Autodesk Inventor part; units mm, degrees
(part 2 of 2)
  point P155 (-22.7596, 134.1998)
  point P156 (-16.0635, 134.1998)
  point P157 (-9.3673, 134.1998)
  point P158 (-2.6712, 134.1998)
  point P159 (-36.1519, 134.1998)
  point P160 (-36.1519, 137.1998)
  point P161 (-32.8038, 140.1998)
  point P162 (-29.4558, 137.1998)
  point P163 (-26.8577, 132.6998)
  point P164 (-26.1077, 140.1998)
  point P165 (-19.4115, 140.1998)
  point P166 (-12.7154, 140.1998)
  point P167 (-6.0192, 140.1998)
  point P168 (-39.5, 140.1998)
  point P169 (-2.5841, 26.25)
  point P170 (-9.2803, 26.25)
  point P171 (-22.6726, 26.25)
  point P172 (-15.9764, 26.25)
  point P173 (-29.3688, 26.25)
  point P174 (-36.0649, 26.25)
  point P175 (-5.9322, 29.25)
  point P176 (0.7639, 29.25)
  point P177 (-29.3688, 29.25)
  point P178 (-22.6726, 29.25)
  point P179 (-19.3245, 29.25)
  point P180 (-12.6284, 29.25)
  point P181 (-26.0207, 29.25)
  point P182 (-32.7168, 29.25)
  point P183 (-2.6712, 14.25)
  point P184 (-9.3673, 14.25)
  point P185 (-22.7596, 14.25)
  point P186 (-16.0635, 14.25)
  point P187 (-29.4558, 14.25)
  point P188 (-36.1519, 14.25)
  point P189 (-6.0192, 17.25)
  point P190 (0.6769, 17.25)
  point P191 (-29.4558, 17.25)
  point P192 (-22.7596, 17.25)
  point P193 (-12.7154, 17.25)
  point P194 (-26.1077, 17.25)
  point P195 (-32.8038, 17.25)
  point P196 (-38.65, 118.709)
  point P197 (-38.65, 113.6905)
  point P198 (-38.65, 137.7905)
  point P199 (-38.65, 17.7407)
  dimension "d0" = 0.35
  dimension "d1" = 2
  constraints: 1624 end point, 3 horizontal, 3 parallel, 3 vertical, 1 perpendicular, 1799 other
  measures "d1" distance between parallel lines of L13 L16
extrude "Extrusión1" add sketch "Boceto1" along normal blind 5 contours L14 L13 L12 L605 L608 L17 L568 L567 L569 L496 L495 L497 L424 L423 L425 L352 L351 L353 L280 L279 L281 L208 L207 L209 L136 L135 L137 L783 L782 L780 L25 L24 L23 L16 L22 L35 L34 L798 L801 L812 L805 L810 L790 L19 L18 L752 L749 L15 | L749 L752 L17 L712 L711 L713 L679 L676 L12 | L676 L679 L17 L680 L677 L12 | L677 L680 L17 L640 L639 L641 L607 L604 L12 | L752 L750 L751 L18 L721 L720 L719 L718 L717 L722 L724 L723 L728 L727 L726 L725 L732 L731 L729 L734 L730 L733 L738 L737 L735 L740 L736 L739 L744 L743 L741 L746 L742 L745 L19 L708 L707 L705 L636 L635 L633 L564 L563 L561 L492 L491 L489 L420 L419 L417 L348 L347 L345 L276 L275 L273 L204 L203 L201 L132 L131 L129 L758 L756 L753 L794 L792 L789 L16 L790 L797 L795 L811 L809 L810 L805 L807 L808 L806 L804 L812 L801 L803 L802 L800 L799 L798 L34 L33 L38 L37 L36 L35 L22 L21 L20 L25 L17 L68 L64 L67 L780 L778 L781 L784 L783 L104 L102 L103 L137 L140 L138 L139 L136 L176 L174 L175 L209 L212 L210 L211 L208 L248 L246 L247 L281 L284 L282 L283 L280 L320 L318 L319 L353 L356 L354 L355 L352 L392 L390 L391 L425 L428 L426 L427 L424 L464 L462 L463 L497 L500 L498 L499 L496 L536 L534 L535 L569 L572 L570 L571 L568 L608 L606 L607 L641 L644 L642 L643 L640 L680 L678 L679 L713 L716 L714 L715 L712 | L604 L607 L17 L608 L605 L12 | L17 L713 L711 L712 | L17 L641 L639 L640 | L17 L569 L567 L568 | L17 L497 L495 L496 | L17 L425 L423 L424 | L17 L353 L351 L352 | L17 L281 L279 L280 | L17 L209 L207 L208 | L17 L137 L135 L136 | L17 L23 L24 L25 | L23 L16 L17 | L16 L22 L23
sketch "Boceto2" plane through (0, 0, 5) normal (0, 0, 1) x (1, 0, 0)
  line L0 (-40.65, 9.35) -> (-1.35, 9.35) projected
  line L1 (-1.35, 9.35) -> (-1.35, 144.35) projected
  line L2 (-1.35, 144.35) -> (-40.65, 144.35) projected
  line L3 (-40.65, 144.35) -> (-40.65, 9.35) projected
  line L4 (-38.65, 118.709) -> (-36.9019, 117.6998) projected
  line L5 (-36.9019, 117.6998) -> (-36.9019, 114.6998) projected
  line L6 (-36.9019, 114.6998) -> (-38.65, 113.6905) projected
  line L7 (-38.65, 113.6905) -> (-38.65, 118.709) projected
  line L8 (-38.65, 137.7905) -> (-38.65, 142.35) projected
  line L9 (-38.65, 142.35) -> (-38.2014, 142.35) projected
  line L10 (-38.2014, 142.35) -> (-36.9885, 141.6498) projected
  line L11 (-36.9885, 141.6498) -> (-36.9885, 138.7498) projected
  line L12 (-36.9885, 138.7498) -> (-38.65, 137.7905) projected
  line L13 (-38.65, 22.7593) -> (-36.9019, 21.75) projected
  line L14 (-36.9019, 21.75) -> (-36.9019, 18.75) projected
  line L15 (-36.9019, 18.75) -> (-38.65, 17.7407) projected
  line L16 (-38.65, 17.7407) -> (-38.65, 22.7593) projected
  line L17 (-38.65, 29.6905) -> (-38.65, 34.709) projected
  line L18 (-38.65, 34.709) -> (-36.9019, 33.6998) projected
  line L19 (-36.9019, 33.6998) -> (-36.9019, 30.6998) projected
  line L20 (-36.9019, 30.6998) -> (-38.65, 29.6905) projected
  line L21 (-38.65, 36.642) -> (-38.65, 39.7575) projected
  line L22 (-38.65, 39.7575) -> (-36.1519, 41.1998) projected
  line L23 (-36.1519, 41.1998) -> (-33.5538, 39.6998) projected
  line L24 (-33.5538, 39.6998) -> (-33.5538, 36.6998) projected
  line L25 (-33.5538, 36.6998) -> (-36.1519, 35.1998) projected
  line L26 (-36.1519, 35.1998) -> (-38.65, 36.642) projected
  line L27 (-38.65, 41.6905) -> (-38.65, 46.709) projected
  line L28 (-38.65, 46.709) -> (-36.9019, 45.6998) projected
  line L29 (-36.9019, 45.6998) -> (-36.9019, 42.6998) projected
  line L30 (-36.9019, 42.6998) -> (-38.65, 41.6905) projected
  line L31 (-38.65, 48.642) -> (-38.65, 51.7575) projected
  line L32 (-38.65, 51.7575) -> (-36.1519, 53.1998) projected
  line L33 (-36.1519, 53.1998) -> (-33.5538, 51.6998) projected
  line L34 (-33.5538, 51.6998) -> (-33.5538, 48.6998) projected
  line L35 (-33.5538, 48.6998) -> (-36.1519, 47.1998) projected
  line L36 (-36.1519, 47.1998) -> (-38.65, 48.642) projected
  line L37 (-38.65, 53.6905) -> (-38.65, 58.709) projected
  line L38 (-38.65, 58.709) -> (-36.9019, 57.6998) projected
  line L39 (-36.9019, 57.6998) -> (-36.9019, 54.6998) projected
  line L40 (-36.9019, 54.6998) -> (-38.65, 53.6905) projected
  line L41 (-38.65, 60.642) -> (-38.65, 63.7575) projected
  line L42 (-38.65, 63.7575) -> (-36.1519, 65.1998) projected
  line L43 (-36.1519, 65.1998) -> (-33.5538, 63.6998) projected
  line L44 (-33.5538, 63.6998) -> (-33.5538, 60.6998) projected
  line L45 (-33.5538, 60.6998) -> (-36.1519, 59.1998) projected
  line L46 (-36.1519, 59.1998) -> (-38.65, 60.642) projected
  line L47 (-38.65, 65.6905) -> (-38.65, 70.709) projected
  line L48 (-38.65, 70.709) -> (-36.9019, 69.6998) projected
  line L49 (-36.9019, 69.6998) -> (-36.9019, 66.6998) projected
  line L50 (-36.9019, 66.6998) -> (-38.65, 65.6905) projected
  line L51 (-38.65, 72.642) -> (-38.65, 75.7575) projected
  line L52 (-38.65, 75.7575) -> (-36.1519, 77.1998) projected
  line L53 (-36.1519, 77.1998) -> (-33.5538, 75.6998) projected
  line L54 (-33.5538, 75.6998) -> (-33.5538, 72.6998) projected
  line L55 (-33.5538, 72.6998) -> (-36.1519, 71.1998) projected
  line L56 (-36.1519, 71.1998) -> (-38.65, 72.642) projected
  line L57 (-38.65, 77.6905) -> (-38.65, 82.709) projected
  line L58 (-38.65, 82.709) -> (-36.9019, 81.6998) projected
  line L59 (-36.9019, 81.6998) -> (-36.9019, 78.6998) projected
  line L60 (-36.9019, 78.6998) -> (-38.65, 77.6905) projected
  line L61 (-38.65, 84.642) -> (-38.65, 87.7575) projected
  line L62 (-38.65, 87.7575) -> (-36.1519, 89.1998) projected
  line L63 (-36.1519, 89.1998) -> (-33.5538, 87.6998) projected
  line L64 (-33.5538, 87.6998) -> (-33.5538, 84.6998) projected
  line L65 (-33.5538, 84.6998) -> (-36.1519, 83.1998) projected
  line L66 (-36.1519, 83.1998) -> (-38.65, 84.642) projected
  line L67 (-38.65, 89.6905) -> (-38.65, 94.709) projected
  line L68 (-38.65, 94.709) -> (-36.9019, 93.6998) projected
  line L69 (-36.9019, 93.6998) -> (-36.9019, 90.6998) projected
  line L70 (-36.9019, 90.6998) -> (-38.65, 89.6905) projected
  line L71 (-38.65, 96.642) -> (-38.65, 99.7575) projected
  line L72 (-38.65, 99.7575) -> (-36.1519, 101.1998) projected
  line L73 (-36.1519, 101.1998) -> (-33.5538, 99.6998) projected
  line L74 (-33.5538, 99.6998) -> (-33.5538, 96.6998) projected
  line L75 (-33.5538, 96.6998) -> (-36.1519, 95.1998) projected
  line L76 (-36.1519, 95.1998) -> (-38.65, 96.642) projected
  line L77 (-38.65, 101.6905) -> (-38.65, 106.709) projected
  line L78 (-38.65, 106.709) -> (-36.9019, 105.6998) projected
  line L79 (-36.9019, 105.6998) -> (-36.9019, 102.6998) projected
  line L80 (-36.9019, 102.6998) -> (-38.65, 101.6905) projected
  line L81 (-38.65, 108.642) -> (-38.65, 111.7575) projected
  line L82 (-38.65, 111.7575) -> (-36.1519, 113.1998) projected
  line L83 (-36.1519, 113.1998) -> (-33.5538, 111.6998) projected
  line L84 (-33.5538, 111.6998) -> (-33.5538, 108.6998) projected
  line L85 (-33.5538, 108.6998) -> (-36.1519, 107.1998) projected
  line L86 (-36.1519, 107.1998) -> (-38.65, 108.642) projected
  line L87 (-38.65, 125.6905) -> (-38.65, 130.709) projected
  line L88 (-38.65, 130.709) -> (-36.9019, 129.6998) projected
  line L89 (-36.9019, 129.6998) -> (-36.9019, 126.6998) projected
  line L90 (-36.9019, 126.6998) -> (-38.65, 125.6905) projected
  line L91 (-38.65, 120.642) -> (-38.65, 123.7575) projected
  line L92 (-38.65, 123.7575) -> (-36.1519, 125.1998) projected
  line L93 (-36.1519, 125.1998) -> (-33.5538, 123.6998) projected
  line L94 (-33.5538, 123.6998) -> (-33.5538, 120.6998) projected
  line L95 (-33.5538, 120.6998) -> (-36.1519, 119.1998) projected
  line L96 (-36.1519, 119.1998) -> (-38.65, 120.642) projected
  line L97 (-38.65, 132.642) -> (-38.65, 135.7575) projected
  line L98 (-38.65, 135.7575) -> (-36.1519, 137.1998) projected
  line L99 (-36.1519, 137.1998) -> (-33.5538, 135.6998) projected
  line L100 (-33.5538, 135.6998) -> (-33.5538, 132.6998) projected
  line L101 (-33.5538, 132.6998) -> (-36.1519, 131.1998) projected
  line L102 (-36.1519, 131.1998) -> (-38.65, 132.642) projected
  line L103 (-34.1025, 142.35) -> (-31.5052, 142.35) projected
  line L104 (-31.5052, 142.35) -> (-30.2924, 141.6498) projected
  line L105 (-30.2924, 141.6498) -> (-30.2924, 138.7498) projected
  line L106 (-30.2924, 138.7498) -> (-32.8038, 137.2998) projected
  line L107 (-32.8038, 137.2998) -> (-35.3153, 138.7498) projected
  line L108 (-35.3153, 138.7498) -> (-35.3153, 141.6498) projected
  line L109 (-35.3153, 141.6498) -> (-34.1025, 142.35) projected
  line L110 (-27.4063, 142.35) -> (-24.8091, 142.35) projected
  line L111 (-24.8091, 142.35) -> (-23.5962, 141.6498) projected
  line L112 (-23.5962, 141.6498) -> (-23.5962, 138.7498) projected
  line L113 (-23.5962, 138.7498) -> (-26.1077, 137.2998) projected
  line L114 (-26.1077, 137.2998) -> (-28.6192, 138.7498) projected
  line L115 (-28.6192, 138.7498) -> (-28.6192, 141.6498) projected
  line L116 (-28.6192, 141.6498) -> (-27.4063, 142.35) projected
  line L117 (-20.7102, 142.35) -> (-18.1129, 142.35) projected
  line L118 (-18.1129, 142.35) -> (-16.9001, 141.6498) projected
  line L119 (-16.9001, 141.6498) -> (-16.9001, 138.7498) projected
  line L120 (-16.9001, 138.7498) -> (-19.4115, 137.2998) projected
  line L121 (-19.4115, 137.2998) -> (-21.923, 138.7498) projected
  line L122 (-21.923, 138.7498) -> (-21.923, 141.6498) projected
  line L123 (-21.923, 141.6498) -> (-20.7102, 142.35) projected
  line L124 (-14.014, 142.35) -> (-11.4168, 142.35) projected
  line L125 (-11.4168, 142.35) -> (-10.2039, 141.6498) projected
  line L126 (-10.2039, 141.6498) -> (-10.2039, 138.7498) projected
  line L127 (-10.2039, 138.7498) -> (-12.7154, 137.2998) projected
  line L128 (-12.7154, 137.2998) -> (-15.2269, 138.7498) projected
  line L129 (-15.2269, 138.7498) -> (-15.2269, 141.6498) projected
  line L130 (-15.2269, 141.6498) -> (-14.014, 142.35) projected
  line L131 (-7.3179, 142.35) -> (-4.7206, 142.35) projected
  line L132 (-4.7206, 142.35) -> (-3.5078, 141.6498) projected
  line L133 (-3.5078, 141.6498) -> (-3.5078, 138.7498) projected
  line L134 (-3.5078, 138.7498) -> (-6.0192, 137.2998) projected
  line L135 (-6.0192, 137.2998) -> (-8.5307, 138.7498) projected
  line L136 (-8.5307, 138.7498) -> (-8.5307, 141.6498) projected
  line L137 (-8.5307, 141.6498) -> (-7.3179, 142.35) projected
  line L138 (-3.35, 136.8078) -> (-3.35, 131.5917) projected
  line L139 (-3.35, 131.5917) -> (-5.2692, 132.6998) projected
  line L140 (-5.2692, 132.6998) -> (-5.2692, 135.6998) projected
  line L141 (-5.2692, 135.6998) -> (-3.35, 136.8078) projected
  line L142 (-3.35, 124.8078) -> (-3.35, 119.5917) projected
  line L143 (-3.35, 119.5917) -> (-5.2692, 120.6998) projected
  line L144 (-5.2692, 120.6998) -> (-5.2692, 123.6998) projected
  line L145 (-5.2692, 123.6998) -> (-3.35, 124.8078) projected
  line L146 (-3.35, 112.8078) -> (-3.35, 107.5917) projected
  line L147 (-3.35, 107.5917) -> (-5.2692, 108.6998) projected
  line L148 (-5.2692, 108.6998) -> (-5.2692, 111.6998) projected
  line L149 (-5.2692, 111.6998) -> (-3.35, 112.8078) projected
  line L150 (-3.35, 100.8078) -> (-3.35, 95.5917) projected
  line L151 (-3.35, 95.5917) -> (-5.2692, 96.6998) projected
  line L152 (-5.2692, 96.6998) -> (-5.2692, 99.6998) projected
  line L153 (-5.2692, 99.6998) -> (-3.35, 100.8078) projected
  line L154 (-3.35, 88.8078) -> (-3.35, 83.5917) projected
  line L155 (-3.35, 83.5917) -> (-5.2692, 84.6998) projected
  line L156 (-5.2692, 84.6998) -> (-5.2692, 87.6998) projected
  line L157 (-5.2692, 87.6998) -> (-3.35, 88.8078) projected
  line L158 (-3.35, 76.8078) -> (-3.35, 71.5917) projected
  line L159 (-3.35, 71.5917) -> (-5.2692, 72.6998) projected
  line L160 (-5.2692, 72.6998) -> (-5.2692, 75.6998) projected
  line L161 (-5.2692, 75.6998) -> (-3.35, 76.8078) projected
  line L162 (-3.35, 64.8078) -> (-3.35, 59.5917) projected
  line L163 (-3.35, 59.5917) -> (-5.2692, 60.6998) projected
  line L164 (-5.2692, 60.6998) -> (-5.2692, 63.6998) projected
  line L165 (-5.2692, 63.6998) -> (-3.35, 64.8078) projected
  line L166 (-3.35, 52.8078) -> (-3.35, 47.5917) projected
  line L167 (-3.35, 47.5917) -> (-5.2692, 48.6998) projected
  line L168 (-5.2692, 48.6998) -> (-5.2692, 51.6998) projected
  line L169 (-5.2692, 51.6998) -> (-3.35, 52.8078) projected
  line L170 (-3.35, 40.8078) -> (-3.35, 35.5917) projected
  line L171 (-3.35, 35.5917) -> (-5.2692, 36.6998) projected
  line L172 (-5.2692, 36.6998) -> (-5.2692, 39.6998) projected
  line L173 (-5.2692, 39.6998) -> (-3.35, 40.8078) projected
  line L174 (-3.35, 28.8078) -> (-3.35, 23.6922) projected
  line L175 (-3.35, 23.6922) -> (-5.1822, 24.75) projected
  line L176 (-5.1822, 24.75) -> (-5.1822, 27.75) projected
  line L177 (-5.1822, 27.75) -> (-3.35, 28.8078) projected
  line L178 (-3.35, 16.8581) -> (-3.35, 11.6419) projected
  line L179 (-3.35, 11.6419) -> (-5.2692, 12.75) projected
  line L180 (-5.2692, 12.75) -> (-5.2692, 15.75) projected
  line L181 (-5.2692, 15.75) -> (-3.35, 16.8581) projected
  line L182 (-9.3673, 11.25) -> (-11.9654, 12.75) projected
  line L183 (-11.9654, 12.75) -> (-11.9654, 15.75) projected
  line L184 (-11.9654, 15.75) -> (-9.3673, 17.25) projected
  line L185 (-9.3673, 17.25) -> (-6.7692, 15.75) projected
  line L186 (-6.7692, 15.75) -> (-6.7692, 12.75) projected
  line L187 (-6.7692, 12.75) -> (-9.3673, 11.25) projected
  line L188 (-16.0635, 11.25) -> (-18.6615, 12.75) projected
  line L189 (-18.6615, 12.75) -> (-18.6615, 15.75) projected
  line L190 (-18.6615, 15.75) -> (-16.0635, 17.25) projected
  line L191 (-16.0635, 17.25) -> (-13.4654, 15.75) projected
  line L192 (-13.4654, 15.75) -> (-13.4654, 12.75) projected
  line L193 (-13.4654, 12.75) -> (-16.0635, 11.25) projected
  line L194 (-22.7596, 11.25) -> (-25.3577, 12.75) projected
  line L195 (-25.3577, 12.75) -> (-25.3577, 15.75) projected
  line L196 (-25.3577, 15.75) -> (-22.7596, 17.25) projected
  line L197 (-22.7596, 17.25) -> (-20.1615, 15.75) projected
  line L198 (-20.1615, 15.75) -> (-20.1615, 12.75) projected
  line L199 (-20.1615, 12.75) -> (-22.7596, 11.25) projected
  line L200 (-29.4558, 11.25) -> (-32.0538, 12.75) projected
  line L201 (-32.0538, 12.75) -> (-32.0538, 15.75) projected
  line L202 (-32.0538, 15.75) -> (-29.4558, 17.25) projected
  line L203 (-29.4558, 17.25) -> (-26.8577, 15.75) projected
  line L204 (-26.8577, 15.75) -> (-26.8577, 12.75) projected
  line L205 (-26.8577, 12.75) -> (-29.4558, 11.25) projected
  line L206 (-36.3251, 11.35) -> (-38.65, 12.6923) projected
  line L207 (-38.65, 12.6923) -> (-38.65, 15.8077) projected
  line L208 (-38.65, 15.8077) -> (-36.1519, 17.25) projected
  line L209 (-36.1519, 17.25) -> (-33.5538, 15.75) projected
  line L210 (-33.5538, 15.75) -> (-33.5538, 12.75) projected
  line L211 (-33.5538, 12.75) -> (-35.9787, 11.35) projected
  line L212 (-9.2803, 29.25) -> (-6.6822, 27.75) projected
  line L213 (-6.6822, 27.75) -> (-6.6822, 24.75) projected
  line L214 (-6.6822, 24.75) -> (-9.2803, 23.25) projected
  line L215 (-9.2803, 23.25) -> (-11.8784, 24.75) projected
  line L216 (-11.8784, 24.75) -> (-11.8784, 27.75) projected
  line L217 (-11.8784, 27.75) -> (-9.2803, 29.25) projected
  line L218 (-18.5745, 24.75) -> (-18.5745, 27.75) projected
  line L219 (-18.5745, 27.75) -> (-15.9764, 29.25) projected
  line L220 (-15.9764, 29.25) -> (-13.3784, 27.75) projected
  line L221 (-13.3784, 27.75) -> (-13.3784, 24.75) projected
  line L222 (-13.3784, 24.75) -> (-15.9764, 23.25) projected
  line L223 (-15.9764, 23.25) -> (-18.5745, 24.75) projected
  line L224 (-22.6726, 23.25) -> (-25.2707, 24.75) projected
  line L225 (-25.2707, 24.75) -> (-25.2707, 27.75) projected
  line L226 (-25.2707, 27.75) -> (-22.6726, 29.25) projected
  line L227 (-22.6726, 29.25) -> (-20.0745, 27.75) projected
  line L228 (-20.0745, 27.75) -> (-20.0745, 24.75) projected
  line L229 (-20.0745, 24.75) -> (-22.6726, 23.25) projected
  line L230 (-29.3688, 23.25) -> (-31.9668, 24.75) projected
  line L231 (-31.9668, 24.75) -> (-31.9668, 27.75) projected
  line L232 (-31.9668, 27.75) -> (-29.3688, 29.25) projected
  line L233 (-29.3688, 29.25) -> (-26.7707, 27.75) projected
  line L234 (-26.7707, 27.75) -> (-26.7707, 24.75) projected
  line L235 (-26.7707, 24.75) -> (-29.3688, 23.25) projected
  line L236 (-36.0649, 23.25) -> (-38.663, 24.75) projected
  line L237 (-38.663, 24.75) -> (-38.663, 27.75) projected
  line L238 (-38.663, 27.75) -> (-36.0649, 29.25) projected
  line L239 (-36.0649, 29.25) -> (-33.4668, 27.75) projected
  line L240 (-33.4668, 27.75) -> (-33.4668, 24.75) projected
  line L241 (-33.4668, 24.75) -> (-36.0649, 23.25) projected
  line L242 (-29.4558, 131.1998) -> (-32.0538, 132.6998) projected
  line L243 (-32.0538, 132.6998) -> (-32.0538, 135.6998) projected
  line L244 (-32.0538, 135.6998) -> (-29.4558, 137.1998) projected
  line L245 (-29.4558, 137.1998) -> (-26.8577, 135.6998) projected
  line L246 (-26.8577, 135.6998) -> (-26.8577, 132.6998) projected
  line L247 (-26.8577, 132.6998) -> (-29.4558, 131.1998) projected
  line L248 (-18.6615, 132.6998) -> (-18.6615, 135.6998) projected
  line L249 (-18.6615, 135.6998) -> (-16.0635, 137.1998) projected
  line L250 (-16.0635, 137.1998) -> (-13.4654, 135.6998) projected
  line L251 (-13.4654, 135.6998) -> (-13.4654, 132.6998) projected
  line L252 (-13.4654, 132.6998) -> (-16.0635, 131.1998) projected
  line L253 (-16.0635, 131.1998) -> (-18.6615, 132.6998) projected
  line L254 (-22.7596, 131.1998) -> (-25.3577, 132.6998) projected
  line L255 (-25.3577, 132.6998) -> (-25.3577, 135.6998) projected
  line L256 (-25.3577, 135.6998) -> (-22.7596, 137.1998) projected
  line L257 (-22.7596, 137.1998) -> (-20.1615, 135.6998) projected
  line L258 (-20.1615, 135.6998) -> (-20.1615, 132.6998) projected
  line L259 (-20.1615, 132.6998) -> (-22.7596, 131.1998) projected
  line L260 (-6.7692, 132.6998) -> (-9.3673, 131.1998) projected
  line L261 (-9.3673, 131.1998) -> (-11.9654, 132.6998) projected
  line L262 (-11.9654, 132.6998) -> (-11.9654, 135.6998) projected
  line L263 (-11.9654, 135.6998) -> (-9.3673, 137.1998) projected
  line L264 (-9.3673, 137.1998) -> (-6.7692, 135.6998) projected
  line L265 (-6.7692, 135.6998) -> (-6.7692, 132.6998) projected
  line L266 (-32.8038, 125.1998) -> (-35.4019, 126.6998) projected
  line L267 (-35.4019, 126.6998) -> (-35.4019, 129.6998) projected
  line L268 (-35.4019, 129.6998) -> (-32.8038, 131.1998) projected
  line L269 (-32.8038, 131.1998) -> (-30.2058, 129.6998) projected
  line L270 (-30.2058, 129.6998) -> (-30.2058, 126.6998) projected
  line L271 (-30.2058, 126.6998) -> (-32.8038, 125.1998) projected
  line L272 (-22.0096, 126.6998) -> (-22.0096, 129.6998) projected
  line L273 (-22.0096, 129.6998) -> (-19.4115, 131.1998) projected
  line L274 (-19.4115, 131.1998) -> (-16.8135, 129.6998) projected
  line L275 (-16.8135, 129.6998) -> (-16.8135, 126.6998) projected
  line L276 (-16.8135, 126.6998) -> (-19.4115, 125.1998) projected
  line L277 (-19.4115, 125.1998) -> (-22.0096, 126.6998) projected
  line L278 (-26.1077, 125.1998) -> (-28.7058, 126.6998) projected
  line L279 (-28.7058, 126.6998) -> (-28.7058, 129.6998) projected
  line L280 (-28.7058, 129.6998) -> (-26.1077, 131.1998) projected
  line L281 (-26.1077, 131.1998) -> (-23.5096, 129.6998) projected
  line L282 (-23.5096, 129.6998) -> (-23.5096, 126.6998) projected
  line L283 (-23.5096, 126.6998) -> (-26.1077, 125.1998) projected
  line L284 (-10.1173, 126.6998) -> (-12.7154, 125.1998) projected
  line L285 (-12.7154, 125.1998) -> (-15.3135, 126.6998) projected
  line L286 (-15.3135, 126.6998) -> (-15.3135, 129.6998) projected
  line L287 (-15.3135, 129.6998) -> (-12.7154, 131.1998) projected
  line L288 (-12.7154, 131.1998) -> (-10.1173, 129.6998) projected
  line L289 (-10.1173, 129.6998) -> (-10.1173, 126.6998) projected
  line L290 (-6.0192, 125.1998) -> (-8.6173, 126.6998) projected
  line L291 (-8.6173, 126.6998) -> (-8.6173, 129.6998) projected
  line L292 (-8.6173, 129.6998) -> (-6.0192, 131.1998) projected
  line L293 (-6.0192, 131.1998) -> (-3.4212, 129.6998) projected
  line L294 (-3.4212, 129.6998) -> (-3.4212, 126.6998) projected
  line L295 (-3.4212, 126.6998) -> (-6.0192, 125.1998) projected
  line L296 (-29.4558, 119.1998) -> (-32.0538, 120.6998) projected
  line L297 (-32.0538, 120.6998) -> (-32.0538, 123.6998) projected
  line L298 (-32.0538, 123.6998) -> (-29.4558, 125.1998) projected
  line L299 (-29.4558, 125.1998) -> (-26.8577, 123.6998) projected
  line L300 (-26.8577, 123.6998) -> (-26.8577, 120.6998) projected
  line L301 (-26.8577, 120.6998) -> (-29.4558, 119.1998) projected
  line L302 (-18.6615, 120.6998) -> (-18.6615, 123.6998) projected
  line L303 (-18.6615, 123.6998) -> (-16.0635, 125.1998) projected
  line L304 (-16.0635, 125.1998) -> (-13.4654, 123.6998) projected
  line L305 (-13.4654, 123.6998) -> (-13.4654, 120.6998) projected
  line L306 (-13.4654, 120.6998) -> (-16.0635, 119.1998) projected
  line L307 (-16.0635, 119.1998) -> (-18.6615, 120.6998) projected
  line L308 (-22.7596, 119.1998) -> (-25.3577, 120.6998) projected
  line L309 (-25.3577, 120.6998) -> (-25.3577, 123.6998) projected
  line L310 (-25.3577, 123.6998) -> (-22.7596, 125.1998) projected
  line L311 (-22.7596, 125.1998) -> (-20.1615, 123.6998) projected
  line L312 (-20.1615, 123.6998) -> (-20.1615, 120.6998) projected
  line L313 (-20.1615, 120.6998) -> (-22.7596, 119.1998) projected
  line L314 (-6.7692, 120.6998) -> (-9.3673, 119.1998) projected
  line L315 (-9.3673, 119.1998) -> (-11.9654, 120.6998) projected
  line L316 (-11.9654, 120.6998) -> (-11.9654, 123.6998) projected
  line L317 (-11.9654, 123.6998) -> (-9.3673, 125.1998) projected
  line L318 (-9.3673, 125.1998) -> (-6.7692, 123.6998) projected
  line L319 (-6.7692, 123.6998) -> (-6.7692, 120.6998) projected
  line L320 (-32.8038, 113.1998) -> (-35.4019, 114.6998) projected
  line L321 (-35.4019, 114.6998) -> (-35.4019, 117.6998) projected
  line L322 (-35.4019, 117.6998) -> (-32.8038, 119.1998) projected
  line L323 (-32.8038, 119.1998) -> (-30.2058, 117.6998) projected
  line L324 (-30.2058, 117.6998) -> (-30.2058, 114.6998) projected
  line L325 (-30.2058, 114.6998) -> (-32.8038, 113.1998) projected
  line L326 (-22.0096, 114.6998) -> (-22.0096, 117.6998) projected
  line L327 (-22.0096, 117.6998) -> (-19.4115, 119.1998) projected
  line L328 (-19.4115, 119.1998) -> (-16.8135, 117.6998) projected
  line L329 (-16.8135, 117.6998) -> (-16.8135, 114.6998) projected
  line L330 (-16.8135, 114.6998) -> (-19.4115, 113.1998) projected
  line L331 (-19.4115, 113.1998) -> (-22.0096, 114.6998) projected
  line L332 (-26.1077, 113.1998) -> (-28.7058, 114.6998) projected
  line L333 (-28.7058, 114.6998) -> (-28.7058, 117.6998) projected
  line L334 (-28.7058, 117.6998) -> (-26.1077, 119.1998) projected
  line L335 (-26.1077, 119.1998) -> (-23.5096, 117.6998) projected
  line L336 (-23.5096, 117.6998) -> (-23.5096, 114.6998) projected
  line L337 (-23.5096, 114.6998) -> (-26.1077, 113.1998) projected
  line L338 (-10.1173, 114.6998) -> (-12.7154, 113.1998) projected
  line L339 (-12.7154, 113.1998) -> (-15.3135, 114.6998) projected
  line L340 (-15.3135, 114.6998) -> (-15.3135, 117.6998) projected
  line L341 (-15.3135, 117.6998) -> (-12.7154, 119.1998) projected
  line L342 (-12.7154, 119.1998) -> (-10.1173, 117.6998) projected
  line L343 (-10.1173, 117.6998) -> (-10.1173, 114.6998) projected
  line L344 (-6.0192, 113.1998) -> (-8.6173, 114.6998) projected
  line L345 (-8.6173, 114.6998) -> (-8.6173, 117.6998) projected
  line L346 (-8.6173, 117.6998) -> (-6.0192, 119.1998) projected
  line L347 (-6.0192, 119.1998) -> (-3.4212, 117.6998) projected
  line L348 (-3.4212, 117.6998) -> (-3.4212, 114.6998) projected
  line L349 (-3.4212, 114.6998) -> (-6.0192, 113.1998) projected
  line L350 (-29.4558, 107.1998) -> (-32.0538, 108.6998) projected
  line L351 (-32.0538, 108.6998) -> (-32.0538, 111.6998) projected
  line L352 (-32.0538, 111.6998) -> (-29.4558, 113.1998) projected
  line L353 (-29.4558, 113.1998) -> (-26.8577, 111.6998) projected
  line L354 (-26.8577, 111.6998) -> (-26.8577, 108.6998) projected
  line L355 (-26.8577, 108.6998) -> (-29.4558, 107.1998) projected
  line L356 (-18.6615, 108.6998) -> (-18.6615, 111.6998) projected
  line L357 (-18.6615, 111.6998) -> (-16.0635, 113.1998) projected
  line L358 (-16.0635, 113.1998) -> (-13.4654, 111.6998) projected
  line L359 (-13.4654, 111.6998) -> (-13.4654, 108.6998) projected
  line L360 (-13.4654, 108.6998) -> (-16.0635, 107.1998) projected
  line L361 (-16.0635, 107.1998) -> (-18.6615, 108.6998) projected
  line L362 (-22.7596, 107.1998) -> (-25.3577, 108.6998) projected
  line L363 (-25.3577, 108.6998) -> (-25.3577, 111.6998) projected
  line L364 (-25.3577, 111.6998) -> (-22.7596, 113.1998) projected
  line L365 (-22.7596, 113.1998) -> (-20.1615, 111.6998) projected
  line L366 (-20.1615, 111.6998) -> (-20.1615, 108.6998) projected
  line L367 (-20.1615, 108.6998) -> (-22.7596, 107.1998) projected
  line L368 (-6.7692, 108.6998) -> (-9.3673, 107.1998) projected
  line L369 (-9.3673, 107.1998) -> (-11.9654, 108.6998) projected
  line L370 (-11.9654, 108.6998) -> (-11.9654, 111.6998) projected
  line L371 (-11.9654, 111.6998) -> (-9.3673, 113.1998) projected
  line L372 (-9.3673, 113.1998) -> (-6.7692, 111.6998) projected
  line L373 (-6.7692, 111.6998) -> (-6.7692, 108.6998) projected
  line L374 (-32.8038, 101.1998) -> (-35.4019, 102.6998) projected
  line L375 (-35.4019, 102.6998) -> (-35.4019, 105.6998) projected
  line L376 (-35.4019, 105.6998) -> (-32.8038, 107.1998) projected
  line L377 (-32.8038, 107.1998) -> (-30.2058, 105.6998) projected
  line L378 (-30.2058, 105.6998) -> (-30.2058, 102.6998) projected
  line L379 (-30.2058, 102.6998) -> (-32.8038, 101.1998) projected
  line L380 (-22.0096, 102.6998) -> (-22.0096, 105.6998) projected
  line L381 (-22.0096, 105.6998) -> (-19.4115, 107.1998) projected
  line L382 (-19.4115, 107.1998) -> (-16.8135, 105.6998) projected
  line L383 (-16.8135, 105.6998) -> (-16.8135, 102.6998) projected
  line L384 (-16.8135, 102.6998) -> (-19.4115, 101.1998) projected
  line L385 (-19.4115, 101.1998) -> (-22.0096, 102.6998) projected
  line L386 (-26.1077, 101.1998) -> (-28.7058, 102.6998) projected
  line L387 (-28.7058, 102.6998) -> (-28.7058, 105.6998) projected
  line L388 (-28.7058, 105.6998) -> (-26.1077, 107.1998) projected
  line L389 (-26.1077, 107.1998) -> (-23.5096, 105.6998) projected
  line L390 (-23.5096, 105.6998) -> (-23.5096, 102.6998) projected
  line L391 (-23.5096, 102.6998) -> (-26.1077, 101.1998) projected
  line L392 (-10.1173, 102.6998) -> (-12.7154, 101.1998) projected
  line L393 (-12.7154, 101.1998) -> (-15.3135, 102.6998) projected
  line L394 (-15.3135, 102.6998) -> (-15.3135, 105.6998) projected
  line L395 (-15.3135, 105.6998) -> (-12.7154, 107.1998) projected
  line L396 (-12.7154, 107.1998) -> (-10.1173, 105.6998) projected
  line L397 (-10.1173, 105.6998) -> (-10.1173, 102.6998) projected
  line L398 (-6.0192, 101.1998) -> (-8.6173, 102.6998) projected
  line L399 (-8.6173, 102.6998) -> (-8.6173, 105.6998) projected
  line L400 (-8.6173, 105.6998) -> (-6.0192, 107.1998) projected
  line L401 (-6.0192, 107.1998) -> (-3.4212, 105.6998) projected
  line L402 (-3.4212, 105.6998) -> (-3.4212, 102.6998) projected
  line L403 (-3.4212, 102.6998) -> (-6.0192, 101.1998) projected
  line L404 (-29.4558, 95.1998) -> (-32.0538, 96.6998) projected
  line L405 (-32.0538, 96.6998) -> (-32.0538, 99.6998) projected
  line L406 (-32.0538, 99.6998) -> (-29.4558, 101.1998) projected
  line L407 (-29.4558, 101.1998) -> (-26.8577, 99.6998) projected
  line L408 (-26.8577, 99.6998) -> (-26.8577, 96.6998) projected
  line L409 (-26.8577, 96.6998) -> (-29.4558, 95.1998) projected
  line L410 (-18.6615, 96.6998) -> (-18.6615, 99.6998) projected
  line L411 (-18.6615, 99.6998) -> (-16.0635, 101.1998) projected
  line L412 (-16.0635, 101.1998) -> (-13.4654, 99.6998) projected
  line L413 (-13.4654, 99.6998) -> (-13.4654, 96.6998) projected
  line L414 (-13.4654, 96.6998) -> (-16.0635, 95.1998) projected
  line L415 (-16.0635, 95.1998) -> (-18.6615, 96.6998) projected
  line L416 (-22.7596, 95.1998) -> (-25.3577, 96.6998) projected
  line L417 (-25.3577, 96.6998) -> (-25.3577, 99.6998) projected
  line L418 (-25.3577, 99.6998) -> (-22.7596, 101.1998) projected
  line L419 (-22.7596, 101.1998) -> (-20.1615, 99.6998) projected
  line L420 (-20.1615, 99.6998) -> (-20.1615, 96.6998) projected
  line L421 (-20.1615, 96.6998) -> (-22.7596, 95.1998) projected
  line L422 (-6.7692, 96.6998) -> (-9.3673, 95.1998) projected
  line L423 (-9.3673, 95.1998) -> (-11.9654, 96.6998) projected
  line L424 (-11.9654, 96.6998) -> (-11.9654, 99.6998) projected
  line L425 (-11.9654, 99.6998) -> (-9.3673, 101.1998) projected
  line L426 (-9.3673, 101.1998) -> (-6.7692, 99.6998) projected
  line L427 (-6.7692, 99.6998) -> (-6.7692, 96.6998) projected
  line L428 (-32.8038, 89.1998) -> (-35.4019, 90.6998) projected
  line L429 (-35.4019, 90.6998) -> (-35.4019, 93.6998) projected
  line L430 (-35.4019, 93.6998) -> (-32.8038, 95.1998) projected
  line L431 (-32.8038, 95.1998) -> (-30.2058, 93.6998) projected
  line L432 (-30.2058, 93.6998) -> (-30.2058, 90.6998) projected
  line L433 (-30.2058, 90.6998) -> (-32.8038, 89.1998) projected
  line L434 (-22.0096, 90.6998) -> (-22.0096, 93.6998) projected
  line L435 (-22.0096, 93.6998) -> (-19.4115, 95.1998) projected
  line L436 (-19.4115, 95.1998) -> (-16.8135, 93.6998) projected
  line L437 (-16.8135, 93.6998) -> (-16.8135, 90.6998) projected
  line L438 (-16.8135, 90.6998) -> (-19.4115, 89.1998) projected
  line L439 (-19.4115, 89.1998) -> (-22.0096, 90.6998) projected
  line L440 (-26.1077, 89.1998) -> (-28.7058, 90.6998) projected
  line L441 (-28.7058, 90.6998) -> (-28.7058, 93.6998) projected
  line L442 (-28.7058, 93.6998) -> (-26.1077, 95.1998) projected
  line L443 (-26.1077, 95.1998) -> (-23.5096, 93.6998) projected
  line L444 (-23.5096, 93.6998) -> (-23.5096, 90.6998) projected
  line L445 (-23.5096, 90.6998) -> (-26.1077, 89.1998) projected
  line L446 (-10.1173, 90.6998) -> (-12.7154, 89.1998) projected
  line L447 (-12.7154, 89.1998) -> (-15.3135, 90.6998) projected
  line L448 (-15.3135, 90.6998) -> (-15.3135, 93.6998) projected
  line L449 (-15.3135, 93.6998) -> (-12.7154, 95.1998) projected
  line L450 (-12.7154, 95.1998) -> (-10.1173, 93.6998) projected
  line L451 (-10.1173, 93.6998) -> (-10.1173, 90.6998) projected
  line L452 (-6.0192, 89.1998) -> (-8.6173, 90.6998) projected
  line L453 (-8.6173, 90.6998) -> (-8.6173, 93.6998) projected
  line L454 (-8.6173, 93.6998) -> (-6.0192, 95.1998) projected
  line L455 (-6.0192, 95.1998) -> (-3.4212, 93.6998) projected
  line L456 (-3.4212, 93.6998) -> (-3.4212, 90.6998) projected
  line L457 (-3.4212, 90.6998) -> (-6.0192, 89.1998) projected
  line L458 (-29.4558, 83.1998) -> (-32.0538, 84.6998) projected
  line L459 (-32.0538, 84.6998) -> (-32.0538, 87.6998) projected
  line L460 (-32.0538, 87.6998) -> (-29.4558, 89.1998) projected
  line L461 (-29.4558, 89.1998) -> (-26.8577, 87.6998) projected
  line L462 (-26.8577, 87.6998) -> (-26.8577, 84.6998) projected
  line L463 (-26.8577, 84.6998) -> (-29.4558, 83.1998) projected
  line L464 (-18.6615, 84.6998) -> (-18.6615, 87.6998) projected
  line L465 (-18.6615, 87.6998) -> (-16.0635, 89.1998) projected
  line L466 (-16.0635, 89.1998) -> (-13.4654, 87.6998) projected
  line L467 (-13.4654, 87.6998) -> (-13.4654, 84.6998) projected
  line L468 (-13.4654, 84.6998) -> (-16.0635, 83.1998) projected
  line L469 (-16.0635, 83.1998) -> (-18.6615, 84.6998) projected
  line L470 (-22.7596, 83.1998) -> (-25.3577, 84.6998) projected
  line L471 (-25.3577, 84.6998) -> (-25.3577, 87.6998) projected
  line L472 (-25.3577, 87.6998) -> (-22.7596, 89.1998) projected
  line L473 (-22.7596, 89.1998) -> (-20.1615, 87.6998) projected
  line L474 (-20.1615, 87.6998) -> (-20.1615, 84.6998) projected
  line L475 (-20.1615, 84.6998) -> (-22.7596, 83.1998) projected
  line L476 (-6.7692, 84.6998) -> (-9.3673, 83.1998) projected
  line L477 (-9.3673, 83.1998) -> (-11.9654, 84.6998) projected
  line L478 (-11.9654, 84.6998) -> (-11.9654, 87.6998) projected
  line L479 (-11.9654, 87.6998) -> (-9.3673, 89.1998) projected
  line L480 (-9.3673, 89.1998) -> (-6.7692, 87.6998) projected
  line L481 (-6.7692, 87.6998) -> (-6.7692, 84.6998) projected
  line L482 (-32.8038, 77.1998) -> (-35.4019, 78.6998) projected
  line L483 (-35.4019, 78.6998) -> (-35.4019, 81.6998) projected
  line L484 (-35.4019, 81.6998) -> (-32.8038, 83.1998) projected
  line L485 (-32.8038, 83.1998) -> (-30.2058, 81.6998) projected
  line L486 (-30.2058, 81.6998) -> (-30.2058, 78.6998) projected
  line L487 (-30.2058, 78.6998) -> (-32.8038, 77.1998) projected
  line L488 (-22.0096, 78.6998) -> (-22.0096, 81.6998) projected
  line L489 (-22.0096, 81.6998) -> (-19.4115, 83.1998) projected
  line L490 (-19.4115, 83.1998) -> (-16.8135, 81.6998) projected
  line L491 (-16.8135, 81.6998) -> (-16.8135, 78.6998) projected
  line L492 (-16.8135, 78.6998) -> (-19.4115, 77.1998) projected
  line L493 (-19.4115, 77.1998) -> (-22.0096, 78.6998) projected
  line L494 (-26.1077, 77.1998) -> (-28.7058, 78.6998) projected
  line L495 (-28.7058, 78.6998) -> (-28.7058, 81.6998) projected
  line L496 (-28.7058, 81.6998) -> (-26.1077, 83.1998) projected
  line L497 (-26.1077, 83.1998) -> (-23.5096, 81.6998) projected
  line L498 (-23.5096, 81.6998) -> (-23.5096, 78.6998) projected
  line L499 (-23.5096, 78.6998) -> (-26.1077, 77.1998) projected
  line L500 (-10.1173, 78.6998) -> (-12.7154, 77.1998) projected
  line L501 (-12.7154, 77.1998) -> (-15.3135, 78.6998) projected
  line L502 (-15.3135, 78.6998) -> (-15.3135, 81.6998) projected
  line L503 (-15.3135, 81.6998) -> (-12.7154, 83.1998) projected
  line L504 (-12.7154, 83.1998) -> (-10.1173, 81.6998) projected
  line L505 (-10.1173, 81.6998) -> (-10.1173, 78.6998) projected
  line L506 (-6.0192, 77.1998) -> (-8.6173, 78.6998) projected
  line L507 (-8.6173, 78.6998) -> (-8.6173, 81.6998) projected
  line L508 (-8.6173, 81.6998) -> (-6.0192, 83.1998) projected
  line L509 (-6.0192, 83.1998) -> (-3.4212, 81.6998) projected
  line L510 (-3.4212, 81.6998) -> (-3.4212, 78.6998) projected
  line L511 (-3.4212, 78.6998) -> (-6.0192, 77.1998) projected
  line L512 (-29.4558, 71.1998) -> (-32.0538, 72.6998) projected
  line L513 (-32.0538, 72.6998) -> (-32.0538, 75.6998) projected
  line L514 (-32.0538, 75.6998) -> (-29.4558, 77.1998) projected
  line L515 (-29.4558, 77.1998) -> (-26.8577, 75.6998) projected
  line L516 (-26.8577, 75.6998) -> (-26.8577, 72.6998) projected
  line L517 (-26.8577, 72.6998) -> (-29.4558, 71.1998) projected
  line L518 (-18.6615, 72.6998) -> (-18.6615, 75.6998) projected
  line L519 (-18.6615, 75.6998) -> (-16.0635, 77.1998) projected
  line L520 (-16.0635, 77.1998) -> (-13.4654, 75.6998) projected
  line L521 (-13.4654, 75.6998) -> (-13.4654, 72.6998) projected
  line L522 (-13.4654, 72.6998) -> (-16.0635, 71.1998) projected
  line L523 (-16.0635, 71.1998) -> (-18.6615, 72.6998) projected
  line L524 (-22.7596, 71.1998) -> (-25.3577, 72.6998) projected
  line L525 (-25.3577, 72.6998) -> (-25.3577, 75.6998) projected
  line L526 (-25.3577, 75.6998) -> (-22.7596, 77.1998) projected
  line L527 (-22.7596, 77.1998) -> (-20.1615, 75.6998) projected
  line L528 (-20.1615, 75.6998) -> (-20.1615, 72.6998) projected
  line L529 (-20.1615, 72.6998) -> (-22.7596, 71.1998) projected
  line L530 (-6.7692, 72.6998) -> (-9.3673, 71.1998) projected
  line L531 (-9.3673, 71.1998) -> (-11.9654, 72.6998) projected
  line L532 (-11.9654, 72.6998) -> (-11.9654, 75.6998) projected
  line L533 (-11.9654, 75.6998) -> (-9.3673, 77.1998) projected
  line L534 (-9.3673, 77.1998) -> (-6.7692, 75.6998) projected
  line L535 (-6.7692, 75.6998) -> (-6.7692, 72.6998) projected
  line L536 (-32.8038, 65.1998) -> (-35.4019, 66.6998) projected
  line L537 (-35.4019, 66.6998) -> (-35.4019, 69.6998) projected
  line L538 (-35.4019, 69.6998) -> (-32.8038, 71.1998) projected
  line L539 (-32.8038, 71.1998) -> (-30.2058, 69.6998) projected
  line L540 (-30.2058, 69.6998) -> (-30.2058, 66.6998) projected
  line L541 (-30.2058, 66.6998) -> (-32.8038, 65.1998) projected
  line L542 (-22.0096, 66.6998) -> (-22.0096, 69.6998) projected
  line L543 (-22.0096, 69.6998) -> (-19.4115, 71.1998) projected
  line L544 (-19.4115, 71.1998) -> (-16.8135, 69.6998) projected
  line L545 (-16.8135, 69.6998) -> (-16.8135, 66.6998) projected
  line L546 (-16.8135, 66.6998) -> (-19.4115, 65.1998) projected
  line L547 (-19.4115, 65.1998) -> (-22.0096, 66.6998) projected
  line L548 (-26.1077, 65.1998) -> (-28.7058, 66.6998) projected
  line L549 (-28.7058, 66.6998) -> (-28.7058, 69.6998) projected
  line L550 (-28.7058, 69.6998) -> (-26.1077, 71.1998) projected
  line L551 (-26.1077, 71.1998) -> (-23.5096, 69.6998) projected
  line L552 (-23.5096, 69.6998) -> (-23.5096, 66.6998) projected
  line L553 (-23.5096, 66.6998) -> (-26.1077, 65.1998) projected
  line L554 (-10.1173, 66.6998) -> (-12.7154, 65.1998) projected
  line L555 (-12.7154, 65.1998) -> (-15.3135, 66.6998) projected
  line L556 (-15.3135, 66.6998) -> (-15.3135, 69.6998) projected
  line L557 (-15.3135, 69.6998) -> (-12.7154, 71.1998) projected
  line L558 (-12.7154, 71.1998) -> (-10.1173, 69.6998) projected
  line L559 (-10.1173, 69.6998) -> (-10.1173, 66.6998) projected
  line L560 (-6.0192, 65.1998) -> (-8.6173, 66.6998) projected
  line L561 (-8.6173, 66.6998) -> (-8.6173, 69.6998) projected
  line L562 (-8.6173, 69.6998) -> (-6.0192, 71.1998) projected
  line L563 (-6.0192, 71.1998) -> (-3.4212, 69.6998) projected
  line L564 (-3.4212, 69.6998) -> (-3.4212, 66.6998) projected
  line L565 (-3.4212, 66.6998) -> (-6.0192, 65.1998) projected
  line L566 (-29.4558, 59.1998) -> (-32.0538, 60.6998) projected
  line L567 (-32.0538, 60.6998) -> (-32.0538, 63.6998) projected
  line L568 (-32.0538, 63.6998) -> (-29.4558, 65.1998) projected
  line L569 (-29.4558, 65.1998) -> (-26.8577, 63.6998) projected
  line L570 (-26.8577, 63.6998) -> (-26.8577, 60.6998) projected
  line L571 (-26.8577, 60.6998) -> (-29.4558, 59.1998) projected
  line L572 (-18.6615, 60.6998) -> (-18.6615, 63.6998) projected
  line L573 (-18.6615, 63.6998) -> (-16.0635, 65.1998) projected
  line L574 (-16.0635, 65.1998) -> (-13.4654, 63.6998) projected
  line L575 (-13.4654, 63.6998) -> (-13.4654, 60.6998) projected
  line L576 (-13.4654, 60.6998) -> (-16.0635, 59.1998) projected
  line L577 (-16.0635, 59.1998) -> (-18.6615, 60.6998) projected
  line L578 (-22.7596, 59.1998) -> (-25.3577, 60.6998) projected
  line L579 (-25.3577, 60.6998) -> (-25.3577, 63.6998) projected
  line L580 (-25.3577, 63.6998) -> (-22.7596, 65.1998) projected
  line L581 (-22.7596, 65.1998) -> (-20.1615, 63.6998) projected
  line L582 (-20.1615, 63.6998) -> (-20.1615, 60.6998) projected
  line L583 (-20.1615, 60.6998) -> (-22.7596, 59.1998) projected
  line L584 (-6.7692, 60.6998) -> (-9.3673, 59.1998) projected
  line L585 (-9.3673, 59.1998) -> (-11.9654, 60.6998) projected
  line L586 (-11.9654, 60.6998) -> (-11.9654, 63.6998) projected
  line L587 (-11.9654, 63.6998) -> (-9.3673, 65.1998) projected
  line L588 (-9.3673, 65.1998) -> (-6.7692, 63.6998) projected
  line L589 (-6.7692, 63.6998) -> (-6.7692, 60.6998) projected
  line L590 (-32.8038, 53.1998) -> (-35.4019, 54.6998) projected
  line L591 (-35.4019, 54.6998) -> (-35.4019, 57.6998) projected
  line L592 (-35.4019, 57.6998) -> (-32.8038, 59.1998) projected
  line L593 (-32.8038, 59.1998) -> (-30.2058, 57.6998) projected
  line L594 (-30.2058, 57.6998) -> (-30.2058, 54.6998) projected
  line L595 (-30.2058, 54.6998) -> (-32.8038, 53.1998) projected
  line L596 (-22.0096, 54.6998) -> (-22.0096, 57.6998) projected
  line L597 (-22.0096, 57.6998) -> (-19.4115, 59.1998) projected
  line L598 (-19.4115, 59.1998) -> (-16.8135, 57.6998) projected
  line L599 (-16.8135, 57.6998) -> (-16.8135, 54.6998) projected
  line L600 (-16.8135, 54.6998) -> (-19.4115, 53.1998) projected
  line L601 (-19.4115, 53.1998) -> (-22.0096, 54.6998) projected
  line L602 (-26.1077, 53.1998) -> (-28.7058, 54.6998) projected
  line L603 (-28.7058, 54.6998) -> (-28.7058, 57.6998) projected
  line L604 (-28.7058, 57.6998) -> (-26.1077, 59.1998) projected
  line L605 (-26.1077, 59.1998) -> (-23.5096, 57.6998) projected
  line L606 (-23.5096, 57.6998) -> (-23.5096, 54.6998) projected
  line L607 (-23.5096, 54.6998) -> (-26.1077, 53.1998) projected
  line L608 (-10.1173, 54.6998) -> (-12.7154, 53.1998) projected
  line L609 (-12.7154, 53.1998) -> (-15.3135, 54.6998) projected
  line L610 (-15.3135, 54.6998) -> (-15.3135, 57.6998) projected
  line L611 (-15.3135, 57.6998) -> (-12.7154, 59.1998) projected
  line L612 (-12.7154, 59.1998) -> (-10.1173, 57.6998) projected
  line L613 (-10.1173, 57.6998) -> (-10.1173, 54.6998) projected
  line L614 (-6.0192, 53.1998) -> (-8.6173, 54.6998) projected
  line L615 (-8.6173, 54.6998) -> (-8.6173, 57.6998) projected
  line L616 (-8.6173, 57.6998) -> (-6.0192, 59.1998) projected
  line L617 (-6.0192, 59.1998) -> (-3.4212, 57.6998) projected
  line L618 (-3.4212, 57.6998) -> (-3.4212, 54.6998) projected
  line L619 (-3.4212, 54.6998) -> (-6.0192, 53.1998) projected
  line L620 (-29.4558, 47.1998) -> (-32.0538, 48.6998) projected
  line L621 (-32.0538, 48.6998) -> (-32.0538, 51.6998) projected
  line L622 (-32.0538, 51.6998) -> (-29.4558, 53.1998) projected
  line L623 (-29.4558, 53.1998) -> (-26.8577, 51.6998) projected
  line L624 (-26.8577, 51.6998) -> (-26.8577, 48.6998) projected
  line L625 (-26.8577, 48.6998) -> (-29.4558, 47.1998) projected
  line L626 (-18.6615, 48.6998) -> (-18.6615, 51.6998) projected
  line L627 (-18.6615, 51.6998) -> (-16.0635, 53.1998) projected
  line L628 (-16.0635, 53.1998) -> (-13.4654, 51.6998) projected
  line L629 (-13.4654, 51.6998) -> (-13.4654, 48.6998) projected
  line L630 (-13.4654, 48.6998) -> (-16.0635, 47.1998) projected
  line L631 (-16.0635, 47.1998) -> (-18.6615, 48.6998) projected
  line L632 (-22.7596, 47.1998) -> (-25.3577, 48.6998) projected
  line L633 (-25.3577, 48.6998) -> (-25.3577, 51.6998) projected
  line L634 (-25.3577, 51.6998) -> (-22.7596, 53.1998) projected
  line L635 (-22.7596, 53.1998) -> (-20.1615, 51.6998) projected
  line L636 (-20.1615, 51.6998) -> (-20.1615, 48.6998) projected
  line L637 (-20.1615, 48.6998) -> (-22.7596, 47.1998) projected
  line L638 (-6.7692, 48.6998) -> (-9.3673, 47.1998) projected
  line L639 (-9.3673, 47.1998) -> (-11.9654, 48.6998) projected
  line L640 (-11.9654, 48.6998) -> (-11.9654, 51.6998) projected
  line L641 (-11.9654, 51.6998) -> (-9.3673, 53.1998) projected
  line L642 (-9.3673, 53.1998) -> (-6.7692, 51.6998) projected
  line L643 (-6.7692, 51.6998) -> (-6.7692, 48.6998) projected
  line L644 (-32.8038, 41.1998) -> (-35.4019, 42.6998) projected
  line L645 (-35.4019, 42.6998) -> (-35.4019, 45.6998) projected
  line L646 (-35.4019, 45.6998) -> (-32.8038, 47.1998) projected
  line L647 (-32.8038, 47.1998) -> (-30.2058, 45.6998) projected
  line L648 (-30.2058, 45.6998) -> (-30.2058, 42.6998) projected
  line L649 (-30.2058, 42.6998) -> (-32.8038, 41.1998) projected
  line L650 (-22.0096, 42.6998) -> (-22.0096, 45.6998) projected
  line L651 (-22.0096, 45.6998) -> (-19.4115, 47.1998) projected
  line L652 (-19.4115, 47.1998) -> (-16.8135, 45.6998) projected
  line L653 (-16.8135, 45.6998) -> (-16.8135, 42.6998) projected
  line L654 (-16.8135, 42.6998) -> (-19.4115, 41.1998) projected
  line L655 (-19.4115, 41.1998) -> (-22.0096, 42.6998) projected
  line L656 (-26.1077, 41.1998) -> (-28.7058, 42.6998) projected
  line L657 (-28.7058, 42.6998) -> (-28.7058, 45.6998) projected
  line L658 (-28.7058, 45.6998) -> (-26.1077, 47.1998) projected
  line L659 (-26.1077, 47.1998) -> (-23.5096, 45.6998) projected
  line L660 (-23.5096, 45.6998) -> (-23.5096, 42.6998) projected
  line L661 (-23.5096, 42.6998) -> (-26.1077, 41.1998) projected
  line L662 (-10.1173, 42.6998) -> (-12.7154, 41.1998) projected
  line L663 (-12.7154, 41.1998) -> (-15.3135, 42.6998) projected
  line L664 (-15.3135, 42.6998) -> (-15.3135, 45.6998) projected
  line L665 (-15.3135, 45.6998) -> (-12.7154, 47.1998) projected
  line L666 (-12.7154, 47.1998) -> (-10.1173, 45.6998) projected
  line L667 (-10.1173, 45.6998) -> (-10.1173, 42.6998) projected
  line L668 (-6.0192, 41.1998) -> (-8.6173, 42.6998) projected
  line L669 (-8.6173, 42.6998) -> (-8.6173, 45.6998) projected
  line L670 (-8.6173, 45.6998) -> (-6.0192, 47.1998) projected
  line L671 (-6.0192, 47.1998) -> (-3.4212, 45.6998) projected
  line L672 (-3.4212, 45.6998) -> (-3.4212, 42.6998) projected
  line L673 (-3.4212, 42.6998) -> (-6.0192, 41.1998) projected
  line L674 (-29.4558, 35.1998) -> (-32.0538, 36.6998) projected
  line L675 (-32.0538, 36.6998) -> (-32.0538, 39.6998) projected
  line L676 (-32.0538, 39.6998) -> (-29.4558, 41.1998) projected
  line L677 (-29.4558, 41.1998) -> (-26.8577, 39.6998) projected
  line L678 (-26.8577, 39.6998) -> (-26.8577, 36.6998) projected
  line L679 (-26.8577, 36.6998) -> (-29.4558, 35.1998) projected
  line L680 (-18.6615, 36.6998) -> (-18.6615, 39.6998) projected
  line L681 (-18.6615, 39.6998) -> (-16.0635, 41.1998) projected
  line L682 (-16.0635, 41.1998) -> (-13.4654, 39.6998) projected
  line L683 (-13.4654, 39.6998) -> (-13.4654, 36.6998) projected
  line L684 (-13.4654, 36.6998) -> (-16.0635, 35.1998) projected
  line L685 (-16.0635, 35.1998) -> (-18.6615, 36.6998) projected
  line L686 (-22.7596, 35.1998) -> (-25.3577, 36.6998) projected
  line L687 (-25.3577, 36.6998) -> (-25.3577, 39.6998) projected
  line L688 (-25.3577, 39.6998) -> (-22.7596, 41.1998) projected
  line L689 (-22.7596, 41.1998) -> (-20.1615, 39.6998) projected
  line L690 (-20.1615, 39.6998) -> (-20.1615, 36.6998) projected
  line L691 (-20.1615, 36.6998) -> (-22.7596, 35.1998) projected
  line L692 (-6.7692, 36.6998) -> (-9.3673, 35.1998) projected
  line L693 (-9.3673, 35.1998) -> (-11.9654, 36.6998) projected
  line L694 (-11.9654, 36.6998) -> (-11.9654, 39.6998) projected
  line L695 (-11.9654, 39.6998) -> (-9.3673, 41.1998) projected
  line L696 (-9.3673, 41.1998) -> (-6.7692, 39.6998) projected
  line L697 (-6.7692, 39.6998) -> (-6.7692, 36.6998) projected
  line L698 (-32.8038, 29.1998) -> (-35.4019, 30.6998) projected
  line L699 (-35.4019, 30.6998) -> (-35.4019, 33.6998) projected
  line L700 (-35.4019, 33.6998) -> (-32.8038, 35.1998) projected
  line L701 (-32.8038, 35.1998) -> (-30.2058, 33.6998) projected
  line L702 (-30.2058, 33.6998) -> (-30.2058, 30.6998) projected
  line L703 (-30.2058, 30.6998) -> (-32.8038, 29.1998) projected
  line L704 (-22.0096, 30.6998) -> (-22.0096, 33.6998) projected
  line L705 (-22.0096, 33.6998) -> (-19.4115, 35.1998) projected
  line L706 (-19.4115, 35.1998) -> (-16.8135, 33.6998) projected
  line L707 (-16.8135, 33.6998) -> (-16.8135, 30.6998) projected
  line L708 (-16.8135, 30.6998) -> (-19.4115, 29.1998) projected
  line L709 (-19.4115, 29.1998) -> (-22.0096, 30.6998) projected
  line L710 (-26.1077, 29.1998) -> (-28.7058, 30.6998) projected
  line L711 (-28.7058, 30.6998) -> (-28.7058, 33.6998) projected
  line L712 (-28.7058, 33.6998) -> (-26.1077, 35.1998) projected
  line L713 (-26.1077, 35.1998) -> (-23.5096, 33.6998) projected
  line L714 (-23.5096, 33.6998) -> (-23.5096, 30.6998) projected
  line L715 (-23.5096, 30.6998) -> (-26.1077, 29.1998) projected
  line L716 (-10.1173, 30.6998) -> (-12.7154, 29.1998) projected
  line L717 (-12.7154, 29.1998) -> (-15.3135, 30.6998) projected
  line L718 (-15.3135, 30.6998) -> (-15.3135, 33.6998) projected
  line L719 (-15.3135, 33.6998) -> (-12.7154, 35.1998) projected
  line L720 (-12.7154, 35.1998) -> (-10.1173, 33.6998) projected
  line L721 (-10.1173, 33.6998) -> (-10.1173, 30.6998) projected
  line L722 (-6.0192, 29.1998) -> (-8.6173, 30.6998) projected
  line L723 (-8.6173, 30.6998) -> (-8.6173, 33.6998) projected
  line L724 (-8.6173, 33.6998) -> (-6.0192, 35.1998) projected
  line L725 (-6.0192, 35.1998) -> (-3.4212, 33.6998) projected
  line L726 (-3.4212, 33.6998) -> (-3.4212, 30.6998) projected
  line L727 (-3.4212, 30.6998) -> (-6.0192, 29.1998) projected
  line L728 (-6.0192, 17.25) -> (-8.6173, 18.75) projected
  line L729 (-8.6173, 18.75) -> (-8.6173, 21.75) projected
  line L730 (-8.6173, 21.75) -> (-6.0192, 23.25) projected
  line L731 (-6.0192, 23.25) -> (-3.4212, 21.75) projected
  line L732 (-3.4212, 21.75) -> (-3.4212, 18.75) projected
  line L733 (-3.4212, 18.75) -> (-6.0192, 17.25) projected
  line L734 (-12.7154, 17.25) -> (-15.3135, 18.75) projected
  line L735 (-15.3135, 18.75) -> (-15.3135, 21.75) projected
  line L736 (-15.3135, 21.75) -> (-12.7154, 23.25) projected
  line L737 (-12.7154, 23.25) -> (-10.1173, 21.75) projected
  line L738 (-10.1173, 21.75) -> (-10.1173, 18.75) projected
  line L739 (-10.1173, 18.75) -> (-12.7154, 17.25) projected
  line L740 (-19.4115, 17.25) -> (-22.0096, 18.75) projected
  line L741 (-22.0096, 18.75) -> (-22.0096, 21.75) projected
  line L742 (-22.0096, 21.75) -> (-19.4115, 23.25) projected
  line L743 (-19.4115, 23.25) -> (-16.8135, 21.75) projected
  line L744 (-16.8135, 21.75) -> (-16.8135, 18.75) projected
  line L745 (-16.8135, 18.75) -> (-19.4115, 17.25) projected
  line L746 (-28.7058, 18.75) -> (-28.7058, 21.75) projected
  line L747 (-28.7058, 21.75) -> (-26.1077, 23.25) projected
  line L748 (-26.1077, 23.25) -> (-23.5096, 21.75) projected
  line L749 (-23.5096, 21.75) -> (-23.5096, 18.75) projected
  line L750 (-23.5096, 18.75) -> (-26.1077, 17.25) projected
  line L751 (-26.1077, 17.25) -> (-28.7058, 18.75) projected
  line L752 (-30.2058, 21.75) -> (-30.2058, 18.75) projected
  line L753 (-30.2058, 18.75) -> (-32.8038, 17.25) projected
  line L754 (-32.8038, 17.25) -> (-35.4019, 18.75) projected
  line L755 (-35.4019, 18.75) -> (-35.4019, 21.75) projected
  line L756 (-35.4019, 21.75) -> (-32.8038, 23.25) projected
  line L757 (-32.8038, 23.25) -> (-30.2058, 21.75) projected
  line L758 (0.15, 7.85) -> (-42.15, 7.85)
  line L759 (-42.15, 7.85) -> (-42.15, 145.85)
  line L760 (-42.15, 145.85) -> (0.15, 145.85)
  line L761 (0.15, 145.85) -> (0.15, 7.85)
  line L762 (-35.9787, 11.35) -> (-36.3251, 11.35) projected
  point P0 (0, 0)
  dimension "d26" = 1.5
  constraints: 8 end point, 3 other
  measures "d26" distance between parallel lines of L0 L758
extrude "Extrusión2" add sketch "Boceto2" against normal blind 2 contours L758 L759 L760 L761
fillet "Empalme1" radius 2 4 edges at (-1.35, 9.35, 1.5) (-40.65, 9.35, 1.5) (-40.65, 144.35, 1.5) (-1.35, 144.35, 1.5)
